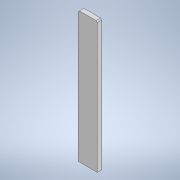
# Autodesk Inventor part: graduated_foot_03
Saved by Autodesk Inventor 2020 (Build 240168000, 168)
## iProperties
Created: 2019-12-19
Part Number: graduated_foot_03
Material: Générique
Document SubType Name: Modeling
Designer: damien
Density: 1 g/cm^3
Appearance: Par défaut
Author: damien
Autodesk Inventor part; units mm, degrees
ref_plane "YZ Plane" through (0, 0, 0) normal (1, 0, 0) x (0, 1, 0)
ref_plane "XZ Plane" through (0, 0, 0) normal (0, 1, 0) x (-1, 0, 0)
ref_plane "XY Plane" through (0, 0, 0) normal (0, 0, 1) x (1, 0, 0)
sketch "Esquisse1" plane through (0, 0, 0) normal (0, 0, 1) x (1, 0, 0)
  line L0 (0, 0) -> (80, 0)
  line L1 (80, 0) -> (80, 550)
  line L2 (80, 550) -> (0, 550)
  line L3 (0, 550) -> (0, 0)
  dimension "d0" = 80
  dimension "d1" = 550
  constraints: 8 end point, 2 parallel, 1 horizontal, 1 perpendicular
  measures "d0" distance of L0.start L0.end
  measures "d1" distance of L2.end L0.start
extrude "Extrusion1" add sketch "Esquisse1" along normal blind 18.55
chamfer "Chanfrein1" distance 5 angle 45 2 edges at (0, 550, 9.275) (80, 550, 9.275)
